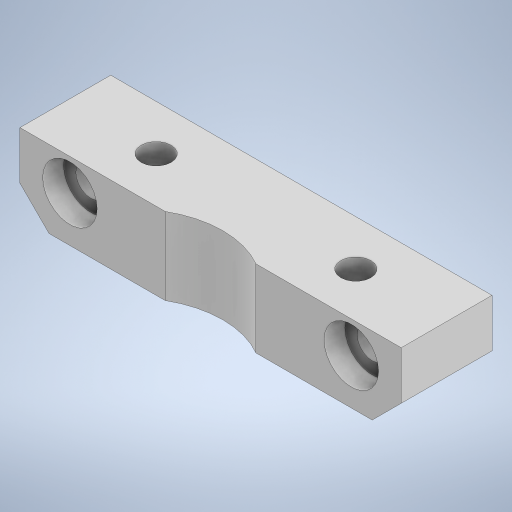
# Autodesk Inventor part: y_motor_lock_bottom1
Saved by Autodesk Inventor 2023 (Build 270158030, 158C)
## iProperties
Created: 2022-05-11
Part Number: y_motor_lock_bottom1
Material: 一般
Document SubType Name: Modeling
Designer: user
Density: 1 g/cm^3
Appearance: 預設
Author: user
## iProperties of the stored document y_motor_lock_bottom1_3D 列印.ipt
Created: 2022-05-15
Part Number: y_motor_lock_bottom1_3D 列印
Material: 一般
Document SubType Name: Modeling
Designer: user
Density: 1 g/cm^3
Appearance: 預設
Author: user
Autodesk Inventor part; units mm, degrees
ref_plane "YZ Plane" through (0, 0, 0) normal (1, 0, 0) x (0, 1, 0)
ref_plane "XZ Plane" through (0, 0, 0) normal (0, 1, 0) x (-1, 0, 0)
ref_plane "XY Plane" through (0, 0, 0) normal (0, 0, 1) x (1, 0, 0)
sketch "草圖1" plane through (0, 0, 0) normal (0, 0, 1) x (1, 0, 0)
  line L0 (-29.4, 0) -> (29.4, 0) projected
  line L1 (0, -5.95) -> (0, 5.95) projected
  line L2 (-21, 4.25) -> (21, 4.25)
  line L3 (21, 4.25) -> (21, -4.25)
  line L4 (21, -4.25) -> (-21, -4.25)
  line L5 (-21, -4.25) -> (-21, 4.25)
  point P0 (0, 0)
  dimension "d0" = 8.5
  dimension "d1" = 42
  constraints: 8 end point, 2 parallel, 1 horizontal, 1 perpendicular, 2 other
  measures "d0" distance of L4.end L2.start
  measures "d1" distance of L2.start L2.end
extrude "擠出1" add sketch "草圖1" along normal blind 10
sketch "草圖2" plane through (-21, -4.25, 0) normal (0, -1, 0) x (1, 0, 0)
  line L0 (0, 0) -> (42, 0) projected
  line L1 (42, 0) -> (42, 10) projected
  line L2 (0, 10) -> (42, 10) projected
  line L3 (0, 0) -> (0, 10) projected
  circle A0 centre (10, 5) radius 4
  circle A1 centre (10, 5) radius 3
  circle A2 centre (10, 5) radius 1.65
  line L4 (21, 0) -> (21, -1.5889)
  circle A3 centre (32, 5) radius 4
  circle A4 centre (32, 5) radius 3
  circle A5 centre (32, 5) radius 1.65
  dimension "d4" = 6
  dimension "d5" = 3.3
  dimension "d6" = 10
  dimension "d29" = 5
  constraints: 6 centre point, 4 coincident, 3 symmetric about line, 2 end point, 1 vertical, 3 other
  measures "d4" diameter of A1
  measures "d5" diameter of A2
  measures "d6" distance from line of L3 A0.centre
  measures "d29" distance from line of L0 A0.centre
extrude "擠出2" cut sketch "草圖2" against normal blind 10 contours A2 | A5
extrude "擠出3" cut sketch "草圖2" against normal blind 2.2 contours A1 | A4
sketch "草圖3" plane through (0, 0, 10) normal (0, 0, 1) x (1, 0, 0)
  line L0 (-21, -4.25) -> (21, -4.25) projected
  line L1 (21, -4.25) -> (21, 4.25) projected
  line L2 (21, 4.25) -> (-21, 4.25) projected
  line L3 (-21, 4.25) -> (-21, -4.25) projected
  line L4 (-17.8, -4.25) -> (-21, -1.05)
  line L5 (0, 4.25) -> (0, 6.2817)
  line L6 (17.8, -4.25) -> (21, -1.05)
  line L7 (17.8, -4.25) -> (22.3255, -4.25) construction
  circle A0 centre (-15.5, 0.75) radius 1.65
  circle A1 centre (-15.5, 0.75) radius 3
  circle A2 centre (15.5, 0.75) radius 1.65
  circle A3 centre (15.5, 0.75) radius 3
  point P0 (0, 0)
  dimension "d11" = 3.2
  dimension "d12" = 45
  dimension "d13" = 45
  dimension "d14" = 3.2
  dimension "d15" = 3.3
  dimension "d16" = 6
  dimension "d17" = 5.5
  dimension "d24" = 3.5
  constraints: 8 end point, 4 centre point, 4 point on line, 2 coincident, 2 symmetric about line, 1 equal length, 1 horizontal, 1 midpoint, 1 vertical, 2 other
  measures "d11" distance from line of L3 L4.start
  measures "d12" angle of L0 L4
  measures "d13" angle of L7 L6
  measures "d14" distance of L0.end L6.start
  measures "d15" diameter of A0
  measures "d16" diameter of A1
  measures "d17" distance from line of L3 A0.centre
  measures "d24" distance from line of L2 A0.centre
extrude "擠出4" cut sketch "草圖3" against normal up to surface (10 mm away) contours L3 L4 L0 | L6 L1 L0 | A0 | A2
extrude "擠出6" cut sketch "草圖3" against normal blind 2.3 contours A1 | A3
sketch "草圖4" plane through (-17.8, -4.25, 0) normal (0, -1, 0) x (1, 0, 0)
  line L0 (0, 10) -> (0, 0) projected
  line L1 (0, 0) -> (35.6, 0) projected
  line L2 (35.6, 0) -> (35.6, 10) projected
  line L3 (0, 10) -> (35.6, 10) projected
  circle A0 centre (28.8, 5) radius 3 projected
  circle A1 centre (6.8, 5) radius 3 projected
  arc A2 (12.8, 10) -> (22.8, 10) centre (17.8, 18.6603) ccw
  line L4 (17.8, 10) -> (17.8, 8.9301)
  point P0 (17.8, 0)
  dimension "d25" = 10
  dimension "d26" = 10
  constraints: 2 end point, 2 point on circle, 2 point on line, 1 centre point, 1 midpoint, 1 symmetric about line, 1 vertical
  measures "d25" radius of A2
  measures "d26" distance of A2.end A2.start
extrude "擠出7" cut sketch "草圖4" against normal up to surface (8.5 mm away) contours L3 A2
equation "\"d27\" = d25"
